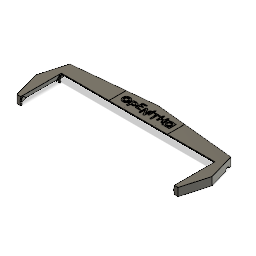
Frame v12 (Autodesk Fusion 360 design; units mm, degrees)
Autodesk Fusion 360 part; units mm, degrees
sketch "Sketch1" plane through (0, 0, 0) normal (0, 1, 0) x (1, 0, 0)
  line L0 (236, 0) -> (236, -125)
  line L1 (236, -125) -> (248, -125)
  line L2 (248, -125) -> (271, -43.5)
  line L3 (271, -43.5) -> (248, 38)
  line L4 (248, 38) -> (0, 63)
  line L5 (0, 63) -> (0, 0)
  line L6 (0, 0) -> (236, 0)
  dimension "d1" = 63
  dimension "d2" = 12
  dimension "d4" = 236
  dimension "d5" = 125
  dimension "d6" = 35
  dimension "d7" = 12
  dimension "d8" = 163
  measures "d1" distance of L5.end
extrude "Extrude1" add sketch "Sketch1" along normal blind 25 makes body 1
sketch "Sketch2" plane through (0, 0, 0) normal (0, -1, 0) x (1, 0, 0)
  line L0 (236, 0) -> (0, 0)
  line L1 (0, 0) -> (0, -63)
  line L2 (0, -63) -> (248, -38)
  line L3 (248, -38) -> (271, 43.5)
  line L4 (271, 43.5) -> (248, 125)
  line L5 (248, 125) -> (236, 125)
  line L6 (236, 125) -> (236, 0)
  line L7 (0, -55) -> (242.0895, -30.5958)
  line L8 (242.0895, -30.5958) -> (263, 43.5)
  line L9 (0, -55) -> (0, 0)
  line L10 (236, 0) -> (0, 0)
  line L11 (236, 0) -> (236, 120)
  line L12 (271, 43.5) -> (263, 43.5) construction
  line L13 (0, -63) -> (0, -55) construction
  line L14 (236, 120) -> (241.411, 120)
  line L15 (241.411, 120) -> (263, 43.5)
  dimension "d11" = 5
  dimension "d12" = 8
  dimension "d13" = 8
extrude "Extrude2" cut sketch "Sketch2" against normal blind 21.5 contours L0 L1 L6 L7 L8 L9 L10 L11 L14 L15 bodies 1
sketch "Sketch3" plane through (0, 0, 0) normal (-1, 0, 0) x (0, 0, 1)
  line L0 (-55, 0) -> (-55, 21.5)
  line L1 (-55, 21.5) -> (0, 21.5)
  line L2 (0, 21.5) -> (0, 25)
  line L3 (0, 25) -> (-63, 25)
  line L4 (-63, 25) -> (-63, 0)
  line L5 (-63, 0) -> (-55, 0)
  circle A0 centre (-22.5958, 0) radius 7
  line L6 (43.5, 0) -> (-30.5958, 0)
  line L7 (-30.5958, 0) -> (-30.5958, 21.5)
  dimension "d16" = 14
  dimension "d18" = 8
  measures "d16" diameter of A0
  measures "d18" distance of origin L7
extrude "Extrude3" cut sketch "Sketch3" against normal through all contours A0 L6 | A0 L6 bodies 1
sketch "Sketch4" plane through (0, 0, 0) normal (0, 0, 1) x (1, 0, 0)
  line L0 (0, 21.5) -> (236, 21.5)
  line L1 (236, 21.5) -> (236, 25)
  line L2 (236, 25) -> (0, 25)
  line L3 (0, 25) -> (0, 21.5)
  line L4 (0, 0) -> (0, 25)
  line L5 (242.0895, 0) -> (0, 0)
  line L6 (0, 0) -> (12, 0)
  line L7 (12, 0) -> (12, 4)
  line L8 (12, 4) -> (0, 4)
  line L9 (0, 4) -> (0, 0)
  arc A0 (12, 4) -> (6, 10) centre (6, 4) ccw
  line L10 (6, 10) -> (0, 10)
  dimension "d104" = 12
  dimension "d105" = 10
  dimension "d106" = 6
  measures "d104" distance of L7 L9
  measures "d105" distance of L6 L10
  measures "d106" radius of A0
extrude "Extrude4" cut sketch "Sketch4" against normal through all contours L4 L5 L6 L7 L8 L9 | L4 L8 A0 L10 bodies 1
sketch "Sketch17" plane through (0, 21.5, 0) normal (0, -1, 0) x (1, 0, 0)
  line L0 (236, 0) -> (0, 0)
  line L1 (0, 0) -> (0, -55)
  line L2 (0, -55) -> (242.0895, -30.5958)
  line L3 (242.0895, -30.5958) -> (263, 43.5)
  line L4 (263, 43.5) -> (241.411, 120)
  line L5 (241.411, 120) -> (236, 120)
  line L6 (236, 120) -> (236, 0)
  line L7 (236, 0) -> (254, 0)
  line L8 (254, 0) -> (254, 5)
  line L9 (254, 5) -> (236, 5)
  line L10 (236, 5) -> (236, 0)
  dimension "d84" = 5
  dimension "d85" = 18
  measures "d84" distance of L0.end
extrude "Extrude15" add sketch "Sketch17" along normal up to surface (21.5 mm away) contours L3 L6 L7 L9 L10 bodies 1
sketch "Sketch18" plane through (0, 0, 0) normal (0, 0, -1) x (-1, 0, 0)
  line L0 (-250.7239, 0) -> (-236, 0)
  line L1 (-236, 0) -> (-236, 21.5)
  line L2 (-236, 21.5) -> (-250.7239, 21.5)
  line L3 (-250.7239, 21.5) -> (-250.7239, 0)
  line L4 (-246, 0) -> (-241, 0)
  line L5 (-241, 0) -> (-241, 8)
  line L6 (-241, 8) -> (-246, 8)
  line L7 (-246, 8) -> (-246, 0)
  arc A0 (-241, 8) -> (-246, 8) centre (-243.5, 8) ccw
  dimension "d88" = 8
  dimension "d89" = 5
  dimension "d90" = 5
  measures "d88" distance of origin
  measures "d89" distance of L1 L5
  measures "d90" distance of L5 L7
extrude "Extrude16" cut sketch "Sketch18" against normal blind 5 contours L0 L4 L5 L6 L7 | L6 A0 bodies 1
mirror "Mirror1" about plane through (0, 0, 0) normal (1, 0, 0) of "Extrude1", "Extrude2", "Extrude3", "Extrude4", "Extrude15", "Extrude16" makes body 2
combine "Combine1" operation add target body 1 tool bodies 2
sketch "Sketch5" plane through (0, 0, 125) normal (0, 0, 1) x (1, 0, 0)
  line L0 (236, 0) -> (248, 0)
  line L1 (248, 0) -> (248, 25)
  line L2 (248, 25) -> (236, 25)
  line L3 (236, 25) -> (236, 0)
  line L4 (242.0895, 0) -> (12, 0)
  line L5 (236, 20) -> (236, 5)
  line L6 (236, 5) -> (234, 10)
  line L7 (234, 10) -> (234, 15)
  line L8 (234, 15) -> (236, 20)
  line L9 (234, 12.5) -> (236, 12.5) construction
  dimension "d59" = 5
  dimension "d60" = 5
  dimension "d61" = 5
  dimension "d62" = 2
  measures "d62" distance of L5 L7
extrude "Extrude5" add sketch "Sketch5" against normal blind 5 bodies 1
sketch "Sketch6" plane through (0, 0, 125) normal (0, 0, 1) x (1, 0, 0)
  line L0 (-248, 0) -> (-236, 0)
  line L1 (-236, 0) -> (-236, 25)
  line L2 (-236, 25) -> (-248, 25)
  line L3 (-248, 25) -> (-248, 0)
  line L4 (-236, 20) -> (-236, 5)
  line L5 (-238, 10) -> (-236, 5)
  line L6 (-238, 10) -> (-238, 15)
  line L7 (-238, 15) -> (-236, 20)
  line L8 (-236, 12.5) -> (-238, 12.5) construction
  dimension "d63" = 5
  dimension "d64" = 5
  dimension "d65" = 5
  dimension "d66" = 2
  measures "d63" distance of origin
  measures "d66" distance of L4 L6
extrude "Extrude6" cut sketch "Sketch6" against normal blind 5 contours L1 L4 L5 L6 L7 bodies 1
ref_plane "WorkPlane1" through (0, 30, 31) normal (0, 1, 0) x (0, 0, 1)
sketch "Sketch8" plane through (0, 21.5, 0) normal (0, -1, 0) x (1, 0, 0)
  line L0 (0, -55) -> (242.0895, -30.5958)
  line L1 (242.0895, -30.5958) -> (250.7239, 0)
  line L2 (236, 0) -> (-236, 0)
  line L3 (-250.7239, 0) -> (-242.0895, -30.5958)
  line L4 (-242.0895, -30.5958) -> (0, -55)
  line L5 (75, -3.4651) -> (-75, -3.4651)
  line L6 (-75, -3.4651) -> (-75, -43.4651)
  line L7 (-75, -43.4651) -> (75, -43.4651)
  line L8 (75, -43.4651) -> (75, -3.4651)
  line L9 (75, -3.4651) -> (-75, -43.4651) construction
  line L10 (-75, -3.4651) -> (75, -43.4651) construction
  line L11 (250.7239, 0) -> (236, 0)
  line L12 (-236, 0) -> (-250.7239, 0)
  dimension "d37" = 150
  dimension "d38" = 40
  measures "d38" distance of origin
sketch "Sketch9" plane through (236, 0, 0) normal (-1, 0, 0) x (0, 0, 1)
  line L0 (125, 20) -> (125, 25)
  line L1 (125, 25) -> (0, 25)
  line L2 (0, 25) -> (0, 21.5)
  line L3 (5, 21.5) -> (120, 21.5)
  line L4 (0, 21.5) -> (7, 21.5)
  line L5 (7, 21.5) -> (14, 13.5)
  line L6 (14, 13.5) -> (109, 13.5)
  line L7 (109, 13.5) -> (116, 21.5)
  line L8 (120, 21.5) -> (120, 20)
  line L9 (120, 20) -> (125, 20)
  line L10 (0, 21.5) -> (0, 0)
  line L11 (0, 0) -> (5, 0)
  line L12 (5, 0) -> (5, 21.5)
  dimension "d41" = 7
  dimension "d43" = 7
  dimension "d44" = 8
  dimension "d45" = 9
  dimension "d46" = 7
  measures "d46" distance of L10.end
extrude "Extrude8" add sketch "Sketch9" against normal blind 3 contours L3 L5 L6 L7 bodies 1
mirror "Mirror2" about plane through (0, 0, 0) normal (1, 0, 0) of "Extrude8"
ref_plane "WorkPlane2" through (90, 0, 0) normal (1, 0, 0) x (0, 1, 0)
split "Split1" by plane through (90, 0, 0) normal (1, 0, 0) bodies 1 makes body 3 at (138.6667, 25, -17.9758)
ref_plane "WorkPlane3" through (-90, 0, 0) normal (1, 0, 0) x (0, 1, 0)
split "Split2" by plane through (-90, 0, 0) normal (1, 0, 0) bodies 1 makes body 4 at (0, 25, -21)
sketch "Sketch10" plane through (0, 21.5, 0) normal (0, -1, 0) x (1, 0, 0)
  line L0 (-90, 0) -> (-90, -45.9274)
  line L1 (-90, -45.9274) -> (0, -55)
  line L2 (0, -55) -> (90, -45.9274)
  line L3 (90, -45.9274) -> (90, 0)
  line L4 (90, 0) -> (-90, 0)
  line L5 (-46.99, -6) -> (46.99, -6) construction
  line L6 (46.99, -6) -> (46.99, -40.29) construction
  line L7 (46.99, -40.29) -> (-46.99, -40.29) construction
  line L8 (-46.99, -40.29) -> (-46.99, -6) construction
  line L9 (0, -40.29) -> (0, -55) construction
  line L10 (-46.99, -40.29) -> (-46.99, -50.2631) construction
  circle A0 centre (-46.99, -6) radius 2.15
  circle A1 centre (46.99, -6) radius 2.15
  circle A2 centre (46.99, -40.29) radius 2.15
  circle A3 centre (-46.99, -40.29) radius 2.15
  dimension "d50" = 93.98
  dimension "d51" = 34.29
  dimension "d52" = 4.3
  dimension "d97" = 6
  measures "d51" distance of origin
  measures "d52" diameter of A1
  measures "d97" distance of L4 L5
extrude "Extrude9" add sketch "Sketch10" along normal blind 3 contours A0 | A1 | A2 | A3 bodies 4
sketch "Sketch11" plane through (0, 18.5, 0) normal (0, -1, 0) x (1, 0, 0)
  circle A0 centre (46.99, -40.29) radius 2.15
  circle A1 centre (46.99, -40.29) radius 2.15
  circle A2 centre (46.99, -6) radius 2.15
  circle A3 centre (-46.99, -40.29) radius 2.15
  circle A4 centre (-46.99, -6) radius 2.15
hole "Hole1" at (46.99, 18.5, -40.29) at (46.99, 18.5, -6) at (-46.99, 18.5, -40.29) at (-46.99, 18.5, -6) direction (0, 1, 0) diameter 1.623 depth 4.5 tip angle 118 bodies 4
thread "Thread1" "ISO Metric profile 2.0 M2x0.4 6H"
sketch "Sketch12" plane through (0, 30, 40.5) normal (0, 1, 0) x (1, 0, 0)
  line L0 (-25.621, 85.9375) -> (-31.3193, 85.8472)
  line L1 (-31.3193, 85.8472) -> (-31.3193, 63.4155)
  line L2 (-31.3193, 63.4155) -> (-23.8722, 63.4486)
  spline S0 degree 3 poles (-23.8722, 63.4486) (-18.8974, 63.4818) (-16.395, 63.5067) (-16.3347, 63.5697) knots 0 0 0 0 1 1 1 1
  spline S1 degree 3 poles (-16.3347, 63.5697) (-16.2741, 63.6278) (-16.7568, 64.1426) (-17.7216, 65.1375) knots 0 0 0 0 1 1 1 1
  line L3 (-17.7216, 65.1375) -> (-19.199, 66.5847)
  line L4 (-19.199, 66.5847) -> (-22.8773, 66.5847)
  spline S2 degree 3 poles (-22.8773, 66.5847) (-25.3497, 66.5847) (-26.3719, 66.5432) (-26.7753, 66.535) knots 0 0 0 0 1 1 1 1
  spline S3 degree 3 poles (-26.7753, 66.535) (-27.2037, 66.5279) (-27.2341, 66.5266) (-27.5205, 66.5847) knots 0 0 0 0 1 1 1 1
  line L5 (-27.5205, 66.5847) -> (-27.5205, 70.2629)
  line L6 (-27.5205, 70.2629) -> (-27.4599, 73.9412)
  line L7 (-27.4599, 73.9412) -> (-19.1686, 73.9412)
  line L8 (-19.1686, 73.9412) -> (-19.1686, 76.9261)
  line L9 (-19.1686, 76.9261) -> (-20.3445, 76.9592)
  spline S4 degree 3 poles (-20.3445, 76.9592) (-21.068, 76.9924) (-22.4248, 76.9592) (-24.3545, 76.9012) knots 0 0 0 0 1 1 1 1
  spline S5 degree 3 poles (-24.3545, 76.9012) (-26.2841, 76.8109) (-27.2791, 76.8109) (-27.3695, 76.9012) knots 0 0 0 0 1 1 1 1
  spline S6 degree 3 poles (-27.3695, 76.9012) (-27.4901, 76.9915) (-27.5504, 77.9866) (-27.5504, 79.9162) knots 0 0 0 0 1 1 1 1
  spline S7 degree 3 poles (-27.5504, 79.9162) (-27.5504, 81.8457) (-27.4899, 82.8408) (-27.3695, 82.9313) knots 0 0 0 0 1 1 1 1
  spline S8 degree 3 poles (-27.3695, 82.9313) (-27.309, 82.9893) (-26.2539, 82.9893) (-24.2339, 82.9644) knots 0 0 0 0 1 1 1 1
  spline S9 degree 3 poles (-24.2339, 82.9644) (-22.0027, 82.9063) (-20.6761, 82.9063) (-20.254, 82.9313) knots 0 0 0 0 1 1 1 1
  line L10 (-20.254, 82.9313) -> (-19.2289, 82.9893)
  line L11 (-19.2289, 82.9893) -> (-17.9325, 84.4366)
  spline S10 degree 3 poles (-17.9325, 84.4366) (-17.0883, 85.4013) (-16.6661, 85.914) (-16.6963, 85.9742) knots 0 0 0 0 1 1 1 1
  spline S11 degree 3 poles (-16.6963, 85.9742) (-16.7867, 86.0073) (-17.3294, 86.0322) (-18.3546, 86.0322) knots 0 0 0 0 1 1 1 1
  spline S12 degree 3 poles (-18.3546, 86.0322) (-18.8973, 85.9991) (-21.3093, 85.9742) (-25.6207, 85.9419) knots 0 0 0 0 1 1 1 1
  line L12 (-25.6207, 85.9419) -> (-25.621, 85.9375)
  spline S13 degree 3 poles (-67.3089, 75.8584) (-68.0324, 75.6777) (-68.6958, 75.3154) (-69.2988, 74.8333) knots 0 0 0 0 1 1 1 1
  spline S14 degree 3 poles (-69.2988, 74.8333) (-69.9017, 74.3211) (-70.3842, 73.748) (-70.6857, 73.145) knots 0 0 0 0 1 1 1 1
  spline S15 degree 3 poles (-70.6857, 73.145) (-71.4696, 71.6375) (-71.4395, 70.0998) (-70.6559, 68.5923) knots 0 0 0 0 1 1 1 1
  spline S16 degree 3 poles (-70.6559, 68.5923) (-69.872, 67.0848) (-68.6358, 66.1803) (-66.9474, 65.9088) knots 0 0 0 0 1 1 1 1
  spline S17 degree 3 poles (-66.9474, 65.9088) (-65.6208, 65.6676) (-64.3846, 65.9669) (-63.239, 66.8134) knots 0 0 0 0 1 1 1 1
  spline S18 degree 3 poles (-63.239, 66.8134) (-62.0932, 67.6274) (-61.3998, 68.7128) (-61.1586, 70.0998) knots 0 0 0 0 1 1 1 1
  spline S19 degree 3 poles (-61.1586, 70.0998) (-60.9174, 71.5469) (-61.2792, 72.8433) (-62.244, 74.0193) knots 0 0 0 0 1 1 1 1
  spline S20 degree 3 poles (-62.244, 74.0193) (-63.2088, 75.1951) (-64.4148, 75.8283) (-65.8922, 75.9187) knots 0 0 0 0 1 1 1 1
  spline S21 degree 3 poles (-65.8922, 75.9187) (-66.5555, 75.9519) (-67.0078, 75.9187) (-67.3092, 75.8607) knots 0 0 0 0 1 1 1 1
  line L13 (-67.3092, 75.8607) -> (-67.3089, 75.8584)
  spline S22 degree 3 poles (-58.5653, 70.8233) (-58.5653, 69.557) (-58.7462, 68.4715) (-59.108, 67.5972) knots 0 0 0 0 1 1 1 1
  spline S23 degree 3 poles (-59.108, 67.5972) (-59.4698, 66.6927) (-60.0427, 65.8787) (-60.8567, 65.125) knots 0 0 0 0 1 1 1 1
  spline S24 degree 3 poles (-60.8567, 65.125) (-62.0325, 63.9793) (-63.4496, 63.316) (-65.0777, 63.105) knots 0 0 0 0 1 1 1 1
  spline S25 degree 3 poles (-65.0777, 63.105) (-66.736, 62.8638) (-68.2737, 63.105) (-69.7209, 63.7988) knots 0 0 0 0 1 1 1 1
  spline S26 degree 3 poles (-69.7209, 63.7988) (-71.1681, 64.4926) (-72.2535, 65.5475) (-72.9168, 66.9344) knots 0 0 0 0 1 1 1 1
  spline S27 degree 3 poles (-72.9168, 66.9344) (-73.5198, 68.1102) (-73.7911, 69.4066) (-73.7911, 70.8238) knots 0 0 0 0 1 1 1 1
  spline S28 degree 3 poles (-73.7911, 70.8238) (-73.7911, 72.8137) (-73.2484, 74.472) (-72.2233, 75.7985) knots 0 0 0 0 1 1 1 1
  spline S29 degree 3 poles (-72.2233, 75.7985) (-71.1982, 77.095) (-69.6907, 77.9694) (-67.731, 78.4216) knots 0 0 0 0 1 1 1 1
  spline S30 degree 3 poles (-67.731, 78.4216) (-67.2486, 78.5417) (-66.5852, 78.5725) (-65.7712, 78.5417) knots 0 0 0 0 1 1 1 1
  spline S31 degree 3 poles (-65.7712, 78.5417) (-64.9873, 78.4837) (-64.2938, 78.3908) (-63.721, 78.2102) knots 0 0 0 0 1 1 1 1
  spline S32 degree 3 poles (-63.721, 78.2102) (-60.2839, 77.1248) (-58.5654, 74.6525) (-58.5653, 70.8233) knots 0 0 0 0 1 1 1 1
  spline S33 degree 3 poles (-67.9118, 81.828) (-69.0576, 81.6473) (-70.1731, 81.285) (-71.3188, 80.7426) knots 0 0 0 0 1 1 1 1
  spline S34 degree 3 poles (-71.3188, 80.7426) (-74.3338, 79.2351) (-76.2634, 76.8231) (-77.0473, 73.5367) knots 0 0 0 0 1 1 1 1
  spline S35 degree 3 poles (-77.0473, 73.5367) (-77.1981, 72.9341) (-77.2584, 72.0292) (-77.2584, 70.8232) knots 0 0 0 0 1 1 1 1
  spline S36 degree 3 poles (-77.2584, 70.8232) (-77.2584, 69.6171) (-77.1978, 68.7127) (-77.0473, 68.1096) knots 0 0 0 0 1 1 1 1
  spline S37 degree 3 poles (-77.0473, 68.1096) (-76.6252, 66.2404) (-75.8715, 64.6423) (-74.7258, 63.2554) knots 0 0 0 0 1 1 1 1
  spline S38 degree 3 poles (-74.7258, 63.2554) (-73.6102, 61.8686) (-72.1931, 60.8434) (-70.5047, 60.1801) knots 0 0 0 0 1 1 1 1
  spline S39 degree 3 poles (-70.5047, 60.1801) (-69.2987, 59.6678) (-67.8817, 59.4266) (-66.2837, 59.4266) knots 0 0 0 0 1 1 1 1
  spline S40 degree 3 poles (-66.2837, 59.4266) (-64.5952, 59.4266) (-63.148, 59.6678) (-61.9119, 60.2108) knots 0 0 0 0 1 1 1 1
  spline S41 degree 3 poles (-61.9119, 60.2108) (-60.1632, 60.9344) (-58.6858, 62.0198) (-57.5401, 63.4369) knots 0 0 0 0 1 1 1 1
  spline S42 degree 3 poles (-57.5401, 63.4369) (-56.3944, 64.8238) (-55.6406, 66.4821) (-55.2487, 68.4117) knots 0 0 0 0 1 1 1 1
  spline S43 degree 3 poles (-55.2487, 68.4117) (-55.1583, 68.9547) (-55.0979, 69.8588) (-55.0979, 71.1252) knots 0 0 0 0 1 1 1 1
  spline S44 degree 3 poles (-55.0979, 71.1252) (-55.0979, 72.3614) (-55.1585, 73.2658) (-55.2788, 73.8085) knots 0 0 0 0 1 1 1 1
  spline S45 degree 3 poles (-55.2788, 73.8085) (-55.7311, 75.8286) (-56.6657, 77.5472) (-58.1129, 78.9341) knots 0 0 0 0 1 1 1 1
  spline S46 degree 3 poles (-58.1129, 78.9341) (-59.5601, 80.321) (-61.339, 81.2254) (-63.4193, 81.6477) knots 0 0 0 0 1 1 1 1
  spline S47 degree 3 poles (-63.4193, 81.6477) (-64.0223, 81.738) (-64.7761, 81.7986) (-65.7409, 81.859) knots 0 0 0 0 1 1 1 1
  spline S48 degree 3 poles (-65.7409, 81.859) (-66.7057, 81.9171) (-67.4293, 81.8922) (-67.9117, 81.8259) knots 0 0 0 0 1 1 1 1
  line L14 (-67.9117, 81.8259) -> (-67.9118, 81.828)
  spline S49 degree 3 poles (-41.0631, 75.1436) (-40.3395, 74.8418) (-39.7364, 74.2693) (-39.3144, 73.4252) knots 0 0 0 0 1 1 1 1
  spline S50 degree 3 poles (-39.3144, 73.4252) (-38.8923, 72.581) (-38.7114, 71.7066) (-38.7717, 70.8321) knots 0 0 0 0 1 1 1 1
  spline S51 degree 3 poles (-38.7717, 70.8321) (-38.8621, 69.9276) (-39.1937, 69.2643) (-39.7666, 68.8422) knots 0 0 0 0 1 1 1 1
  spline S52 degree 3 poles (-39.7666, 68.8422) (-40.3696, 68.3897) (-41.0631, 68.0887) (-41.9073, 67.9076) knots 0 0 0 0 1 1 1 1
  spline S53 degree 3 poles (-41.9073, 67.9076) (-42.7515, 67.7269) (-43.9274, 67.6365) (-45.465, 67.6365) knots 0 0 0 0 1 1 1 1
  line L15 (-45.465, 67.6365) -> (-47.6962, 67.6365)
  line L16 (-47.6962, 67.6365) -> (-47.6962, 75.3249)
  line L17 (-47.6962, 75.3249) -> (-44.5907, 75.3249)
  spline S54 degree 3 poles (-44.5907, 75.3249) (-42.5405, 75.3249) (-41.3646, 75.2668) (-41.0631, 75.1436) knots 0 0 0 0 1 1 1 1
  line L18 (-52.0377, 56.3601) -> (-47.5755, 56.3601)
  line L19 (-47.5755, 56.3601) -> (-47.5755, 64.1389)
  line L20 (-47.5755, 64.1389) -> (-45.7966, 64.197)
  spline S55 degree 3 poles (-45.7966, 64.197) (-42.9625, 64.3171) (-40.9123, 64.5583) (-39.646, 64.8907) knots 0 0 0 0 1 1 1 1
  spline S56 degree 3 poles (-39.646, 64.8907) (-38.3797, 65.1925) (-37.3244, 65.765) (-36.5104, 66.549) knots 0 0 0 0 1 1 1 1
  spline S57 degree 3 poles (-36.5104, 66.549) (-35.3646, 67.6947) (-34.6712, 69.2323) (-34.4903, 71.2222) knots 0 0 0 0 1 1 1 1
  spline S58 degree 3 poles (-34.4903, 71.2222) (-34.3094, 73.2123) (-34.7013, 74.8101) (-35.636, 76.0464) knots 0 0 0 0 1 1 1 1
  spline S59 degree 3 poles (-35.636, 76.0464) (-35.9073, 76.3779) (-36.2993, 76.7095) (-36.8118, 77.0714) knots 0 0 0 0 1 1 1 1
  spline S60 degree 3 poles (-36.8118, 77.0714) (-37.3545, 77.4337) (-37.8972, 77.7048) (-38.4399, 77.9156) knots 0 0 0 0 1 1 1 1
  spline S61 degree 3 poles (-38.4399, 77.9156) (-39.4651, 78.2779) (-40.3997, 78.5182) (-41.2439, 78.6094) knots 0 0 0 0 1 1 1 1
  spline S62 degree 3 poles (-41.2439, 78.6094) (-42.0881, 78.6997) (-43.9273, 78.7603) (-46.7916, 78.7902) knots 0 0 0 0 1 1 1 1
  line L21 (-46.7916, 78.7902) -> (-52.0377, 78.8233)
  line L22 (-52.0377, 78.8233) -> (-52.0377, 56.3601)
  line L23 (1.5198, 77.0344) -> (-0.1083, 75.4062)
  spline S63 degree 3 poles (-0.1083, 75.4062) (-0.1083, 73.9591) (-0.1382, 71.7881) (-0.1382, 68.8938) knots 0 0 0 0 1 1 1 1
  spline S64 degree 3 poles (-0.1382, 68.8938) (-0.168, 65.9994) (-0.168, 63.8286) (-0.168, 62.3815) knots 0 0 0 0 1 1 1 1
  line L24 (-0.168, 62.3815) -> (-0.4997, 62.9543)
  spline S65 degree 3 poles (-0.4997, 62.9543) (-0.6203, 63.1351) (-1.0424, 64.07) (-1.766, 65.7282) knots 0 0 0 0 1 1 1 1
  spline S66 degree 3 poles (-1.766, 65.7282) (-2.3087, 66.9945) (-3.4243, 69.3764) (-5.0524, 72.9341) knots 0 0 0 0 1 1 1 1
  spline S67 degree 3 poles (-5.0524, 72.9341) (-6.7106, 76.4616) (-7.585, 78.2707) (-7.6453, 78.3611) knots 0 0 0 0 1 1 1 1
  spline S68 degree 3 poles (-7.6453, 78.3611) (-7.7058, 78.3942) (-8.6101, 78.4192) (-10.4191, 78.4192) knots 0 0 0 0 1 1 1 1
  line L25 (-10.4191, 78.4192) -> (-13.0723, 78.386)
  spline S69 degree 3 poles (-13.0723, 78.386) (-13.0723, 75.9137) (-13.1022, 72.2354) (-13.1022, 67.3511) knots 0 0 0 0 1 1 1 1
  spline S70 degree 3 poles (-13.1022, 67.3511) (-13.132, 62.4667) (-13.132, 58.7884) (-13.132, 56.3462) knots 0 0 0 0 1 1 1 1
  line L26 (-13.132, 56.3462) -> (-9.7854, 56.3462)
  line L27 (-9.7854, 56.3462) -> (-9.7854, 65.4516)
  line L28 (-9.7854, 65.4516) -> (-9.7555, 74.5267)
  line L29 (-9.7555, 74.5267) -> (-9.2731, 73.5318)
  spline S71 degree 3 poles (-9.2731, 73.5318) (-8.7003, 72.3559) (-7.8561, 70.6072) (-6.7707, 68.2555) knots 0 0 0 0 1 1 1 1
  spline S72 degree 3 poles (-6.7707, 68.2555) (-5.836, 66.2052) (-5.1426, 64.7278) (-4.6602, 63.8234) knots 0 0 0 0 1 1 1 1
  spline S73 degree 3 poles (-4.6602, 63.8234) (-4.2079, 62.9189) (-3.6049, 61.6827) (-2.821, 60.1149) knots 0 0 0 0 1 1 1 1
  line L30 (-2.821, 60.1149) -> (-1.0723, 56.3462)
  line L31 (-1.0723, 56.3462) -> (3.4804, 56.3462)
  line L32 (3.4804, 56.3462) -> (3.4804, 67.5319)
  spline S74 degree 3 poles (3.4804, 67.5319) (3.4804, 74.9488) (3.4198, 78.6874) (3.3296, 78.6874) knots 0 0 0 0 1 1 1 1
  spline S75 degree 3 poles (3.3296, 78.6874) (3.209, 78.6874) (2.606, 78.1146) (1.5205, 77.0292) knots 0 0 0 0 1 1 1 1
  line L33 (1.5205, 77.0292) -> (1.5198, 77.0344)
  line L34 (8.3945, 84.3002) -> (6.6156, 82.5515)
  line L35 (6.6156, 82.5515) -> (6.5858, 72.994)
  line L36 (6.5858, 72.994) -> (6.5858, 63.4362)
  line L37 (6.5858, 63.4362) -> (10.3847, 63.4362)
  line L38 (10.3847, 63.4362) -> (10.3847, 74.7124)
  spline S76 degree 3 poles (10.3847, 74.7124) (10.3847, 82.25) (10.3242, 86.0188) (10.2641, 86.0188) knots 0 0 0 0 1 1 1 1
  spline S77 degree 3 poles (10.2641, 86.0188) (10.1435, 86.0188) (9.5405, 85.446) (8.3945, 84.3002) knots 0 0 0 0 1 1 1 1
  line L39 (13.4866, 75.7141) -> (17.587, 75.7141)
  spline S78 degree 3 poles (17.587, 75.7141) (20.3006, 75.7141) (21.6875, 75.656) (21.6875, 75.5939) knots 0 0 0 0 1 1 1 1
  spline S79 degree 3 poles (21.6875, 75.5939) (21.6875, 75.5608) (21.5668, 75.3826) (21.3257, 75.0816) knots 0 0 0 0 1 1 1 1
  spline S80 degree 3 poles (21.3257, 75.0816) (21.1147, 74.8404) (20.8734, 74.5088) (20.6322, 74.0867) knots 0 0 0 0 1 1 1 1
  line L40 (20.6322, 74.0867) -> (20.3006, 73.5138)
  line L41 (20.3006, 73.5138) -> (20.3006, 56.3583)
  line L42 (20.3006, 56.3583) -> (24.1598, 56.3583)
  line L43 (24.1598, 56.3583) -> (24.1598, 75.7141)
  line L44 (24.1598, 75.7141) -> (30.8531, 75.7141)
  line L45 (30.8531, 75.7141) -> (30.8531, 78.9402)
  line L46 (30.8531, 78.9402) -> (13.4866, 78.9402)
  line L47 (13.4866, 78.9402) -> (13.4866, 75.7141)
  line L48 (35.7365, 83.505) -> (33.9576, 81.7865)
  line L49 (33.9576, 81.7865) -> (33.9576, 63.0632)
  line L50 (33.9576, 63.0632) -> (37.8169, 63.0632)
  line L51 (37.8169, 63.0632) -> (37.8169, 70.6309)
  spline S81 degree 3 poles (37.8169, 70.6309) (38.8419, 70.6309) (40.3796, 70.5978) (42.4298, 70.5978) knots 0 0 0 0 1 1 1 1
  spline S82 degree 3 poles (42.4298, 70.5978) (44.4801, 70.5646) (46.0177, 70.5646) (47.0428, 70.5646) knots 0 0 0 0 1 1 1 1
  spline S83 degree 3 poles (47.0428, 70.5646) (47.0428, 69.7204) (47.0759, 68.4843) (47.0759, 66.826) knots 0 0 0 0 1 1 1 1
  spline S84 degree 3 poles (47.0759, 66.826) (47.0759, 65.1376) (47.0759, 63.9015) (47.1091, 63.0573) knots 0 0 0 0 1 1 1 1
  line L52 (47.1091, 63.0573) -> (50.9683, 63.0573)
  line L53 (50.9683, 63.0573) -> (50.9683, 74.1526)
  spline S85 degree 3 poles (50.9683, 74.1526) (50.9683, 81.5394) (50.9102, 85.2479) (50.8174, 85.2479) knots 0 0 0 0 1 1 1 1
  spline S86 degree 3 poles (50.8174, 85.2479) (50.6972, 85.2479) (50.0639, 84.675) (48.9179, 83.5595) knots 0 0 0 0 1 1 1 1
  line L54 (48.9179, 83.5595) -> (47.1691, 81.8409)
  spline S87 degree 3 poles (47.1691, 81.8409) (47.1691, 80.9967) (47.136, 79.7002) (47.1111, 78.0119) knots 0 0 0 0 1 1 1 1
  spline S88 degree 3 poles (47.1111, 78.0119) (47.078, 76.2934) (47.053, 74.9969) (47.053, 74.1527) knots 0 0 0 0 1 1 1 1
  line L55 (47.053, 74.1527) -> (37.8874, 74.1527)
  line L56 (37.8874, 74.1527) -> (37.8293, 79.7004)
  spline S89 degree 3 poles (37.8293, 79.7004) (37.7962, 83.3786) (37.7389, 85.248) (37.6486, 85.248) knots 0 0 0 0 1 1 1 1
  spline S90 degree 3 poles (37.6486, 85.248) (37.5284, 85.248) (36.8951, 84.6454) (35.7492, 83.4993) knots 0 0 0 0 1 1 1 1
  line L57 (35.7492, 83.4993) -> (35.7365, 83.505)
  spline S91 degree 3 poles (64.3396, 75.3156) (63.3447, 75.0446) (62.5004, 74.5314) (61.8371, 73.8082) knots 0 0 0 0 1 1 1 1
  spline S92 degree 3 poles (61.8371, 73.8082) (61.1739, 73.0845) (60.7216, 72.1801) (60.5406, 71.1551) knots 0 0 0 0 1 1 1 1
  spline S93 degree 3 poles (60.5406, 71.1551) (60.3897, 70.3708) (60.4502, 69.5872) (60.7213, 68.8033) knots 0 0 0 0 1 1 1 1
  spline S94 degree 3 poles (60.7213, 68.8033) (60.9625, 67.9892) (61.3845, 67.2958) (61.9574, 66.753) knots 0 0 0 0 1 1 1 1
  spline S95 degree 3 poles (61.9574, 66.753) (62.9222, 65.7882) (64.0378, 65.2756) (65.3342, 65.2154) knots 0 0 0 0 1 1 1 1
  spline S96 degree 3 poles (65.3342, 65.2154) (66.6005, 65.1574) (67.7462, 65.5172) (68.7713, 66.3008) knots 0 0 0 0 1 1 1 1
  spline S97 degree 3 poles (68.7713, 66.3008) (69.7663, 67.0851) (70.3994, 68.1701) (70.6406, 69.5269) knots 0 0 0 0 1 1 1 1
  spline S98 degree 3 poles (70.6406, 69.5269) (70.8213, 70.6123) (70.6406, 71.6977) (70.0976, 72.7229) knots 0 0 0 0 1 1 1 1
  spline S99 degree 3 poles (70.0976, 72.7229) (69.5547, 73.748) (68.7408, 74.5017) (67.6856, 75.0142) knots 0 0 0 0 1 1 1 1
  spline S100 degree 3 poles (67.6856, 75.0142) (66.6001, 75.4967) (65.4846, 75.5871) (64.3396, 75.3156) knots 0 0 0 0 1 1 1 1
  spline S101 degree 3 poles (67.5355, 77.8784) (68.5907, 77.6671) (69.5555, 77.2451) (70.46, 76.6122) knots 0 0 0 0 1 1 1 1
  spline S102 degree 3 poles (70.46, 76.6122) (71.3646, 75.949) (72.0278, 75.2252) (72.4499, 74.381) knots 0 0 0 0 1 1 1 1
  spline S103 degree 3 poles (72.4499, 74.381) (72.9323, 73.4162) (73.2034, 72.2101) (73.2941, 70.8233) knots 0 0 0 0 1 1 1 1
  spline S104 degree 3 poles (73.2941, 70.8233) (73.3522, 69.0143) (73.0529, 67.4765) (72.3293, 66.1802) knots 0 0 0 0 1 1 1 1
  spline S105 degree 3 poles (72.3293, 66.1802) (71.6056, 64.8536) (70.5203, 63.8586) (69.0731, 63.1651) knots 0 0 0 0 1 1 1 1
  spline S106 degree 3 poles (69.0731, 63.1651) (66.6913, 62.0193) (64.3094, 62.0193) (61.9275, 63.1651) knots 0 0 0 0 1 1 1 1
  spline S107 degree 3 poles (61.9275, 63.1651) (61.2644, 63.4669) (60.631, 63.9493) (60.0281, 64.552) knots 0 0 0 0 1 1 1 1
  spline S108 degree 3 poles (60.0281, 64.552) (59.4254, 65.1546) (58.9427, 65.7581) (58.6411, 66.4212) knots 0 0 0 0 1 1 1 1
  spline S109 degree 3 poles (58.6411, 66.4212) (58.0982, 67.567) (57.8271, 68.8635) (57.8271, 70.2805) knots 0 0 0 0 1 1 1 1
  spline S110 degree 3 poles (57.8271, 70.2805) (57.8271, 71.6675) (58.0982, 72.9337) (58.6411, 74.0492) knots 0 0 0 0 1 1 1 1
  spline S111 degree 3 poles (58.6411, 74.0492) (59.6663, 76.0995) (61.4752, 77.4261) (64.0078, 77.9687) knots 0 0 0 0 1 1 1 1
  spline S112 degree 3 poles (64.0078, 77.9687) (65.0631, 78.1801) (66.239, 78.1495) (67.5355, 77.8784) knots 0 0 0 0 1 1 1 1
  spline S113 degree 3 poles (63.6461, 81.4362) (62.8321, 81.316) (61.9577, 81.044) (61.023, 80.6519) knots 0 0 0 0 1 1 1 1
  spline S114 degree 3 poles (61.023, 80.6519) (60.0582, 80.23) (59.3044, 79.8078) (58.7015, 79.3556) knots 0 0 0 0 1 1 1 1
  line L58 (58.7015, 79.3556) -> (58.0076, 78.8433)
  spline S115 degree 3 poles (58.0076, 78.8433) (57.9745, 78.8433) (57.6462, 79.024) (57.0127, 79.4459) knots 0 0 0 0 1 1 1 1
  spline S116 degree 3 poles (57.0127, 79.4459) (56.3495, 79.8678) (55.7162, 80.2599) (55.0831, 80.6518) knots 0 0 0 0 1 1 1 1
  spline S117 degree 2 poles (55.0831, 80.6518) (54.4199, 81.0439) (54.0882, 81.2247) knots 0 0 0 1 1 1
  spline S118 degree 3 poles (54.0882, 81.2247) (54.0301, 81.1666) (53.9978, 77.456) (53.9978, 70.1294) knots 0 0 0 0 1 1 1 1
  line L59 (53.9978, 70.1294) -> (54.0309, 59.1547)
  line L60 (54.0309, 59.1547) -> (57.7696, 59.1547)
  line L61 (57.7696, 59.1547) -> (57.8028, 60.3005)
  spline S119 degree 3 poles (57.8028, 60.3005) (57.8028, 61.0847) (57.8359, 61.4763) (57.8931, 61.4763) knots 0 0 0 0 1 1 1 1
  line L62 (57.8931, 61.4763) -> (58.7674, 60.843)
  spline S120 degree 3 poles (58.7674, 60.843) (60.275, 59.6672) (62.0236, 58.9737) (63.9834, 58.7325) knots 0 0 0 0 1 1 1 1
  spline S121 degree 3 poles (63.9834, 58.7325) (65.5211, 58.5212) (67.0587, 58.6124) (68.5662, 59.0343) knots 0 0 0 0 1 1 1 1
  spline S122 degree 3 poles (68.5662, 59.0343) (70.0738, 59.4563) (71.4003, 60.1197) (72.5159, 61.0543) knots 0 0 0 0 1 1 1 1
  line L63 (72.5159, 61.0543) -> (73.2098, 61.5974)
  spline S123 degree 3 poles (73.2098, 61.5974) (73.2098, 61.2956) (73.2429, 60.8737) (73.2429, 60.301) knots 0 0 0 0 1 1 1 1
  spline S124 degree 3 poles (73.2429, 60.301) (73.2429, 59.7281) (73.2429, 59.306) (73.2761, 59.0347) knots 0 0 0 0 1 1 1 1
  spline S125 degree 3 poles (73.2761, 59.0347) (73.6375, 59.0347) (74.2408, 59.0016) (75.0248, 59.0016) knots 0 0 0 0 1 1 1 1
  spline S126 degree 3 poles (75.0248, 59.0016) (75.8089, 58.9684) (76.3816, 58.9684) (76.8036, 58.9684) knots 0 0 0 0 1 1 1 1
  line L64 (76.8036, 58.9684) -> (76.8036, 70.1542)
  spline S127 degree 3 poles (76.8036, 70.1542) (76.8036, 77.5712) (76.7705, 81.3097) (76.7456, 81.3097) knots 0 0 0 0 1 1 1 1
  spline S128 degree 3 poles (76.7456, 81.3097) (76.6875, 81.3097) (76.2632, 81.0685) (75.4189, 80.6159) knots 0 0 0 0 1 1 1 1
  spline S129 degree 3 poles (75.4189, 80.6159) (74.5747, 80.1335) (73.9717, 79.8018) (73.6702, 79.6209) knots 0 0 0 0 1 1 1 1
  spline S130 degree 3 poles (73.6702, 79.6209) (73.3386, 79.3797) (73.1273, 79.2894) (73.0369, 79.2894) knots 0 0 0 0 1 1 1 1
  spline S131 degree 3 poles (73.0369, 79.2894) (72.9167, 79.2894) (72.6149, 79.4403) (72.1023, 79.8017) knots 0 0 0 0 1 1 1 1
  spline S132 degree 3 poles (72.1023, 79.8017) (71.0771, 80.4649) (69.841, 80.9474) (68.454, 81.249) knots 0 0 0 0 1 1 1 1
  spline S133 degree 3 poles (68.454, 81.249) (67.8514, 81.3691) (67.037, 81.4297) (66.0119, 81.4902) knots 0 0 0 0 1 1 1 1
  spline S134 degree 3 poles (66.0119, 81.4902) (64.9867, 81.5233) (64.2029, 81.4902) (63.6602, 81.4321) knots 0 0 0 0 1 1 1 1
  line L65 (63.6602, 81.4321) -> (63.6461, 81.4362)
split_face "SplitFace13" 1 faces at (0, 25, -21) by curves path "Sketch12" along S21 L13 S13 S14 S15 S16 S17 S18 S19 S20 on bodies 4
split_face "SplitFace14" 1 faces at (9.331, 25, -30.1744) by curves path "Sketch12" along S32 S22 S23 S24 S25 S26 S27 S28 S29 S30 S31 on bodies 4
split_face "SplitFace15" 1 faces at (10.1282, 25, -29.7002) by curves path "Sketch12" along S47 S48 L14 S33 S34 S35 S36 S37 S38 S39 S40 S41 S42 S43 S44 S45 S46 on bodies 4
split_face "SplitFace16" 1 faces at (11.1963, 25, -29.2063) by curves path "Sketch12" along S50 S51 S52 S53 L15 L16 L17 S54 S49 on bodies 4
split_face "SplitFace17" 1 faces at (60, 25, -38.9758) by curves path "Sketch12" along L18 L19 L20 S55 S56 S57 S58 S59 S60 S61 S62 L21 L22 on bodies 4
split_face "SplitFace18" 1 faces at (60, 25, -38.9758) by curves path "Sketch12" along L2 S0 S1 L3 L4 S2 S3 L5 L6 L7 L8 L9 S4 S5 S6 S7 S8 S9 L10 L11 S10 S11 S12 L12 L0 L1 on bodies 4
split_face "SplitFace19" 1 faces at (60, 25, -38.9758) by curves path "Sketch12" along L25 S69 S70 L26 L27 L28 L29 S71 S72 S73 L30 L31 L32 S74 S75 L33 L23 S63 S64 L24 S65 S66 S67 S68 on bodies 4
split_face "SplitFace20" 1 faces at (61.1601, 25, -26.9865) by curves path "Sketch12" along L34 L35 L36 L37 L38 S76 S77 on bodies 4
split_face "SplitFace21" 1 faces at (63.4616, 25, -25.6212) by curves path "Sketch12" along L39 S78 S79 S80 L40 L41 L42 L43 L44 L45 L46 L47 on bodies 4
split_face "SplitFace22" 1 faces at (70.2844, 25, -29.7138) by curves path "Sketch12" along S90 L57 L48 L49 L50 L51 S81 S82 S83 S84 L52 L53 S85 S86 L54 S87 S88 L55 L56 S89 on bodies 4
split_face "SplitFace23" 1 faces at (76.9894, 25, -25.4949) by curves path "Sketch12" along S92 S93 S94 S95 S96 S97 S98 S99 S100 S91 on bodies 4
split_face "SplitFace24" 1 faces at (83.5666, 25, -27.8265) by curves path "Sketch12" along S103 S104 S105 S106 S107 S108 S109 S110 S111 S112 S101 S102 on bodies 4
split_face "SplitFace25" 1 faces at (-0.3574, 25, -5.2821) by curves path "Sketch12" along L65 S113 S114 L58 S115 S116 S117 S118 L59 L60 L61 S119 L62 S120 S121 S122 L63 S123 S124 S125 S126 L64 S127 S128 S129 S130 S131 S132 S133 S134 on bodies 4
move_face "OffsetFaces2" offset -0.6 10 faces at (-56.3116, 25, -29.3678) (-65.1701, 25, -31.4074) (-50.5906, 25, -27.1067) (-30.0329, 25, -33.9013) (2.2642, 25, -21.5865) (9.1184, 25, -29.8809) (22.8734, 25, -28.0288) (35.244, 25, -31.3269) (55.3073, 25, -23.0868) (63.9448, 25, -30.8787) on bodies 4
sketch "Sketch19" plane through (0, 0, 5) normal (0, 0, 1) x (1, 0, 0)
  line L0 (241, 0) -> (241, 8)
  arc A0 (246, 8) -> (241, 8) centre (243.5, 8) ccw
  line L1 (246, 8) -> (246, 0)
  line L2 (246, 0) -> (252.135, 0)
  line L3 (252.135, 0) -> (252.135, 21.5)
  line L4 (252.135, 21.5) -> (236, 21.5)
  line L5 (236, 21.5) -> (236, 0)
  line L6 (236, 0) -> (241, 0)
  line L7 (234, 15) -> (236, 20)
  line L8 (234, 10) -> (234, 15)
  line L9 (236, 5) -> (234, 10)
extrude "Extrude17" add sketch "Sketch19" against normal blind 5 contours L5 L7 L8 L9 bodies 3
sketch "Sketch20" plane through (0, 0, 5) normal (0, 0, 1) x (1, 0, 0)
  line L0 (-241, 8) -> (-241, 0)
  line L1 (-241, 0) -> (-236, 0)
  line L2 (-236, 0) -> (-236, 21.5)
  line L3 (-236, 21.5) -> (-252.135, 21.5)
  line L4 (-252.135, 21.5) -> (-252.135, 0)
  line L5 (-252.135, 0) -> (-246, 0)
  line L6 (-246, 0) -> (-246, 8)
  arc A0 (-241, 8) -> (-246, 8) centre (-243.5, 8) ccw
  line L7 (-238, 15) -> (-236, 20)
  line L8 (-238, 10) -> (-238, 15)
  line L9 (-236, 5) -> (-238, 10)
extrude "Extrude18" cut sketch "Sketch20" against normal blind 5 contours L2 L7 L8 L9 bodies 1
sketch "Sketch21" plane through (0, 0, 0) normal (0, -1, 0) x (1, 0, 0)
  line L0 (-12, -55) -> (12, -55)
  line L1 (12, -55) -> (12, -53.7903)
  line L2 (12, -53.7903) -> (-12, -53.7903)
  line L3 (-12, -53.7903) -> (-12, -55)
  line L4 (-246, 0) -> (-246, 5)
  line L5 (-246, 5) -> (-252.135, 5)
  line L6 (-252.135, 5) -> (-263, 43.5)
  line L7 (-263, 43.5) -> (-241.411, 120)
  line L8 (-241.411, 120) -> (-236, 120)
  line L9 (-236, 120) -> (-236, 125)
  line L10 (-236, 125) -> (-248, 125)
  line L11 (-248, 125) -> (-271, 43.5)
  line L12 (-271, 43.5) -> (-254.3227, -15.5958)
  line L13 (-254.3227, -15.5958) -> (-246.3227, -15.5958)
  line L14 (-246.3227, -15.5958) -> (-250.7239, 0)
  line L15 (-250.7239, 0) -> (-246, 0)
  line L16 (-241, 5) -> (-241, 0)
  line L17 (-241, 0) -> (-236, 0)
  line L18 (-236, 0) -> (-236, 5)
  line L19 (-236, 5) -> (-241, 5)
extrude "Extrude19" cut sketch "Sketch21" against normal up to surface (21.5 mm away) contours L0 L1 L2 L3 bodies 4
sketch "Sketch22" plane through (0, 0, -55) normal (0, 0, 1) x (1, 0, 0)
  line L0 (12, 4) -> (12, 21.5)
  line L1 (12, 21.5) -> (-12, 21.5)
  line L2 (-12, 21.5) -> (-12, 4)
  circle A0 centre (0, 10) radius 3
  circle A1 centre (0, 10) radius 7.5
  arc A2 (-6, 10) -> (-12, 4) centre (-6, 4) ccw
  line L3 (-6, 10) -> (6, 10)
  arc A3 (12, 4) -> (6, 10) centre (6, 4) ccw
  dimension "d100" = 6
  dimension "d101" = 15
  measures "d100" diameter of A0
  measures "d101" diameter of A1
extrude "Extrude20" cut sketch "Sketch22" against normal blind 4 contours A0 A1 A2 L3 A3 picked at (5.1714, 11.4803) bodies 4
equation "d39 = ( 180 / 2 ) * 1 mm"
equation "d40 = ( -180 / 2 ) * 1 mm"
named bodies: "Left Frame", "Right Frame", "Center Frame"
